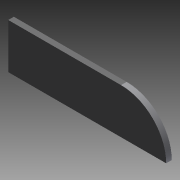
# Autodesk Inventor part: lexan stuff
Saved by Autodesk Inventor 2011 (Build 150239000, 239)
## iProperties
Created: 2013-01-27
Part Number: lexan stuff
Document SubType Name: Modeling
Designer: Danny
Density: 1 g/cm^3
Author: Danny
Autodesk Inventor part; units mm, degrees
ref_plane "YZ Plane" through (0, 0, 0) normal (1, 0, 0) x (0, 1, 0)
ref_plane "XZ Plane" through (0, 0, 0) normal (0, 1, 0) x (-1, 0, 0)
ref_plane "XY Plane" through (0, 0, 0) normal (0, 0, 1) x (1, 0, 0)
sketch "Sketch1" plane through (0, 0, 0) normal (0, 0, 1) x (1, 0, 0)
  line L0 (0, 0) -> (-177.8, 0)
  line L1 (-177.8, 0) -> (-177.8, 50.8)
  line L2 (-177.8, 50.8) -> (-50.8, 50.8)
  line L3 (0, 0) -> (0, 0)
  arc A0 (0, 47.625) -> (-3.175, 50.8) centre (-3.175, 47.625) ccw
  arc A1 (0, 47.625) -> (-3.175, 50.8) centre (-3.175, 47.625) ccw
  arc A2 (0, 0) -> (-50.8, 50.8) centre (-50.8, 0) ccw
  point P0 (0, 50.8)
  dimension "d0" = 177.8
  dimension "d1" = 50.8
  dimension "d4" = 3.175
  dimension "d5" = 50.8
  constraints: 8 end point, 6 point on circle, 6 point on line, 6 tangent, 3 centre point, 2 parallel, 1 concentric, 1 horizontal, 1 perpendicular
  measures "d0" distance of L1.end point (0, 50.8)
  measures "d1" distance of L0.end L1.end
  measures "d4" radius of A0
  measures "d5" radius of A2
extrude "Extrusion1" add sketch "Sketch1" along normal blind 6.35
body "Solid1"
